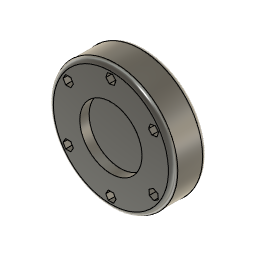
7-rolima_entre_a_garra_e_a_conexao_punho_garra v1 (Autodesk Fusion 360 design; units mm, degrees)
Autodesk Fusion 360 part; units mm, degrees
sketch "Sketch1" plane through (0, 0, 0) normal (0, 1, 0) x (1, 0, 0)
  circle A0 centre (0, 0) radius 10
  circle A1 centre (0, 0) radius 20
  circle A2 centre (0, 0) radius 18.0278 construction
  circle A3 centre (-0.0049, -16.3778) radius 1.65
  line L0 (0, -22) -> (0, 22) construction
  line L1 (-25, 0) -> (28, 0) construction
  circle A4 centre (-0.0049, 16.3778) radius 1.65
  circle A5 centre (0, 0) radius 10
  circle A6 centre (13.7352, 8.9204) radius 1.65
  circle A7 centre (13.7352, -8.9204) radius 1.65
  circle A8 centre (0, 0) radius 10
  circle A9 centre (-13.7352, 8.9204) radius 1.65
  circle A10 centre (-13.7352, -8.9204) radius 1.65
  line L2 (-12.0852, -8.9204) -> (-12.9102, -7.4915)
  line L3 (-12.9102, -7.4915) -> (-14.5602, -7.4915)
  line L4 (-14.5602, -7.4915) -> (-15.3852, -8.9204)
  line L5 (-15.3852, -8.9204) -> (-14.5602, -10.3494)
  line L6 (-14.5602, -10.3494) -> (-12.9102, -10.3494)
  line L7 (-12.9102, -10.3494) -> (-12.0852, -8.9204)
  line L8 (1.1004, -15.1527) -> (-0.5132, -14.808)
  line L9 (-0.5132, -14.808) -> (-1.6185, -16.033)
  line L10 (-1.6185, -16.033) -> (-1.1102, -17.6028)
  line L11 (-1.1102, -17.6028) -> (0.5034, -17.9475)
  line L12 (0.5034, -17.9475) -> (1.6087, -16.7225)
  line L13 (1.6087, -16.7225) -> (1.1004, -15.1527)
  line L14 (14.8062, -7.6652) -> (13.1837, -7.3653)
  line L15 (13.1837, -7.3653) -> (12.1127, -8.6205)
  line L16 (12.1127, -8.6205) -> (12.6643, -10.1756)
  line L17 (12.6643, -10.1756) -> (14.2868, -10.4755)
  line L18 (14.2868, -10.4755) -> (15.3578, -9.2203)
  line L19 (15.3578, -9.2203) -> (14.8062, -7.6652)
  line L20 (12.3594, 9.8312) -> (12.2586, 8.1842)
  line L21 (12.2586, 8.1842) -> (13.6345, 7.2735)
  line L22 (13.6345, 7.2735) -> (15.1111, 8.0097)
  line L23 (15.1111, 8.0097) -> (15.2119, 9.6566)
  line L24 (15.2119, 9.6566) -> (13.836, 10.5673)
  line L25 (13.836, 10.5673) -> (12.3594, 9.8312)
  line L26 (1.6451, 16.3778) -> (0.8201, 17.8067)
  line L27 (0.8201, 17.8067) -> (-0.8299, 17.8067)
  line L28 (-0.8299, 17.8067) -> (-1.6549, 16.3778)
  line L29 (-1.6549, 16.3778) -> (-0.8299, 14.9488)
  line L30 (-0.8299, 14.9488) -> (0.8201, 14.9488)
  line L31 (0.8201, 14.9488) -> (1.6451, 16.3778)
  line L32 (-12.0852, 8.9204) -> (-12.9102, 10.3494)
  line L33 (-12.9102, 10.3494) -> (-14.5602, 10.3494)
  line L34 (-14.5602, 10.3494) -> (-15.3852, 8.9204)
  line L35 (-15.3852, 8.9204) -> (-14.5602, 7.4915)
  line L36 (-14.5602, 7.4915) -> (-12.9102, 7.4915)
  line L37 (-12.9102, 7.4915) -> (-12.0852, 8.9204)
  point P0 (-13.7352, -8.9204)
  point P1 (-0.0049, -16.3778)
  point P2 (13.7352, -8.9204)
  point P3 (13.7352, 8.9204)
  point P4 (-0.0049, 16.3778)
  point P5 (-13.7352, 8.9204)
  dimension "d1" = 20
  dimension "d2" = 40
  dimension "d3" = 3.3
  dimension "d4" = 3.3
  constraint coincident A0.centre A1.centre
  constraint concentric A1 A2
  constraint tangent A2 A3
  constraint vertical L0
  constraint horizontal L1
  constraint symmetric A0 L1 A5
  constraint symmetric A3 L1 A4
  constraint tangent A2 A6
  constraint symmetric L1 A5 A8
  constraint symmetric L1 A6 A7
  constraint symmetric L0 A6 A9
  constraint symmetric L0 A7 A10
  constraint coincident A10 L2.start
  constraint coincident P0 A10.centre
  constraint coincident P1 A3.centre
  constraint coincident A3 L8.start
  constraint coincident A7 L14.start
  constraint coincident P2 A7.centre
  constraint coincident P3 A6.centre
  constraint coincident A6 L20.start
  constraint coincident P4 A4.centre
  constraint coincident A4 L26.start
  constraint coincident P5 A9.centre
  constraint coincident A9 L32.start
  measures "d1" diameter of A0
  measures "d2" diameter of A1
  measures "d3" diameter of A3
  measures "d4" diameter of A6
extrude "Extrude1" add sketch "Sketch1" along normal blind 11 contours A0 A5 A8 | A1 | A3 L13 | A3 L8 | L8 L9 L10 L11 L12 L13 | A3 L12 | A3 L9 | A3 L11 | A3 L10 | A4 L26 | L26 L27 L28 L29 L30 L31 | A4 L31 | A4 L27 | A4 L30 | A4 L28 | A4 L29 | A6 L23 | A6 L24 | L20 L21 L22 L23 L24 L25 | A6 L22 | A6 L25 | A6 L21 | A6 L20 | A7 L19 | A7 L14 | L14 L15 L16 L17 L18 L19 | A7 L18 | A7 L15 | A7 L17 | A7 L16 | A9 L32 | L32 L33 L34 L35 L36 L37 | A9 L37 | A9 L33 | A9 L36 | A9 L34 | A9 L35 | A10 L2 | L2 L3 L4 L5 L6 L7 | A10 L7 | A10 L3 | A10 L6 | A10 L4 | A10 L5
extrude "Extrude2" cut sketch "Sketch1" along normal blind 8 contours L8 L9 L10 L11 L12 L13 | L26 L27 L28 L29 L30 L31 | L20 L21 L22 L23 L24 L25 | L14 L15 L16 L17 L18 L19 | L32 L33 L34 L35 L36 L37 | L2 L3 L4 L5 L6 L7
extrude "Extrude3" cut sketch "Sketch1" along normal blind 3 contours A0 A5 A8
fillet "Fillet1" radius 1.5 2 edges at (-18.6465, 0, 7.2323) (-18.6465, 11, 7.2323)
